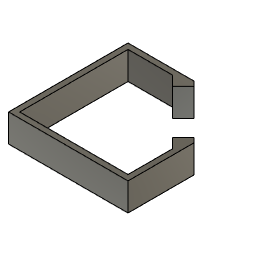
_RoomLayout.3ade8614-bf8f-4f98-9b3b-9bac14557cd1 (Autodesk Fusion 360 design; units mm, degrees)
Autodesk Fusion 360 part; units mm, degrees
sketch "Sketch1" plane through (0, 0, 0) normal (0, 0, 1) x (1, 0, 0)
  line L0 (0, 0) -> (0, 990.6)
  line L1 (0, 990.6) -> (406.4, 990.6)
  line L2 (406.4, 990.6) -> (990.6, 406.4)
  line L3 (990.6, 406.4) -> (990.6, 0)
  line L4 (990.6, 0) -> (0, 0)
  line L5 (-50.8, 1041.4) -> (1041.4, 1041.4)
  line L6 (1041.4, 1041.4) -> (1041.4, -50.8)
  line L7 (1041.4, -50.8) -> (-50.8, -50.8)
  line L8 (-50.8, -50.8) -> (-50.8, 1041.4)
  line L9 (496.2026, 900.7974) -> (636.8051, 1041.4)
  line L10 (900.7974, 496.2026) -> (1041.4, 636.8051)
  line L11 (496.2026, 900.7974) -> (45.8038, 450.3987) construction
  line L12 (45.8038, 450.3987) -> (496.2026, 0) construction
  line L13 (553.1656, 1041.4) -> (1041.4, 553.1656)
  dimension "d1" = 990.6
  dimension "d2" = 990.6
  dimension "d3" = 135
  dimension "d4" = 406.4
  dimension "d5" = 50.8
  dimension "d6" = 50.8
  dimension "d7" = 50.8
  dimension "d8" = 50.8
  dimension "d9" = 127
  dimension "d10" = 127
  dimension "d13" = 139.7
  constraint coincident L0.start L4.end
  constraint vertical L0
  constraint perpendicular L0 L1
  constraint perpendicular L1 L3
  constraint perpendicular L3 L4
  constraint horizontal L5
  constraint vertical L6
  constraint horizontal L7
  constraint vertical L8
  constraint coincident L2 L9.start
  constraint coincident L5 L9.end
  constraint perpendicular L2 L9
  constraint coincident L2 L10.start
  constraint coincident L6 L10.end
  constraint perpendicular L2 L10
  constraint perpendicular L2 L11
  constraint coincident L4 L12.end
  constraint perpendicular L11 L12
  constraint coincident L11.end L12.start
  constraint equal L11 L12
  constraint coincident L5 L13.start
  constraint coincident L6 L13.end
  constraint perpendicular L10 L13
  measures "d1" distance of L3.end L0.start
  measures "d2" distance of L0.start L0.end
  measures "d3" angle of L2 L3
  measures "d4" distance of L2.end L3.end
  measures "d5" distance of L4 L7
  measures "d6" distance of L0 L8
  measures "d7" distance of L3 L6
  measures "d8" distance of L1 L5
  measures "d9" distance of L2.end L10
  measures "d10" distance of L1.end L9
  measures "d13" distance of L2 L13
extrude "Extrude1" add sketch "Sketch1" along normal blind 254 contours L0 L1 L2 L3 L4 L5 L6 L7 L8 L9 L10 L13
